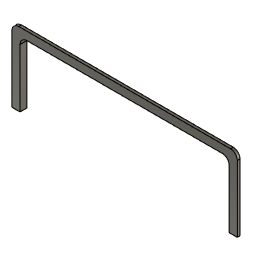
Fysetc_5i_LCD_Door Bezel (Autodesk Fusion 360 design; units mm, degrees)
Autodesk Fusion 360 part; units mm, degrees
sketch "Sketch1" plane through (0, 0, 0) normal (0, 1, 0) x (1, 0, 0)
  line L0 (0, 0) -> (158, 0)
  line L1 (158, 0) -> (158, -50)
  line L2 (158, -50) -> (0, -50)
  line L3 (0, -50) -> (0, 0)
  line L4 (2, 0) -> (156, 0)
  line L5 (156, 0) -> (156, -48)
  line L6 (156, -48) -> (2, -48)
  line L7 (2, -48) -> (2, 0)
  line L8 (-4, 0) -> (162, 0)
  line L9 (162, 0) -> (162, -54)
  line L10 (162, -54) -> (-4, -54)
  line L11 (-4, -54) -> (-4, 0)
  dimension "d1" = 158
  dimension "d2" = 50
  dimension "d3" = 2
  dimension "d4" = 2
  dimension "d5" = 2
  dimension "d6" = 4
  dimension "d7" = 4
  dimension "d8" = 4
  constraint horizontal L0
  constraint vertical L1
  constraint horizontal L2
  constraint vertical L3
  constraint coincident L0.start L3.end
  constraint horizontal L4
  constraint vertical L5
  constraint horizontal L6
  constraint vertical L7
  constraint coincident L0 L4.start
  constraint horizontal L8
  constraint vertical L9
  constraint horizontal L10
  constraint vertical L11
  constraint coincident L0.start L8
  measures "d1" distance of L0.start L0.end
  measures "d2" distance of L0.start L2.end
  measures "d3" distance of L1 L5
  measures "d4" distance of L2 L6
  measures "d5" distance of L3 L7
  measures "d6" distance of L1 L9
  measures "d7" distance of L3 L11
  measures "d8" distance of L2 L10
extrude "Extrude1" add sketch "Sketch1" along normal blind 3 contours L0 L1 L2 L3 L5 L6 L7 L8
extrude "Extrude2" add sketch "Sketch1" against normal blind 2 contours L0 L1 L2 L3 L5 L6 L7 L8 | L1 L2 L3 L8 L9 L10 L11
fillet "Fillet1" radius 5 6 edges at (2, 0.5, 48) (156, 0.5, 48) (158, 1.5, 50) (162, -1, 54) (0, 1.5, 50) (-4, -1, 54)
equation "d4 = d3"
equation "d5 = d4"
equation "d7 = d6"
equation "d8 = d6"
